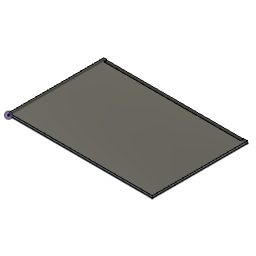
Clear Nomad 3 - Top Panel (Autodesk Fusion 360 design; units mm, degrees)
Autodesk Fusion 360 part; units mm, degrees
note: some values were not read from the file. Set by a fixed rule: which sketch regions a step uses.
sketch "Sketch1" plane through (0, 0, 0) normal (0, 0, 1) x (1, 0, 0)
  line L0 (0, 0) -> (417, 0)
  line L1 (417, 0) -> (417, 276)
  line L2 (0, 276) -> (0, 0)
  line L3 (0, 276) -> (417, 276)
  dimension "d1" = 417
  dimension "d2" = 276
  constraint horizontal L0
  constraint vertical L1
  constraint vertical L2
  constraint coincident L0.start L2.end
  constraint horizontal L3
  measures "d1" distance of L0.start L0.end
  measures "d2" distance of L0.start L2.start
extrude "Extrude1" add sketch "Sketch1" along normal blind 6
sketch "Sketch2" plane through (0, 0, 6) normal (0, 0, 1) x (-1, 0, 0)
  line L0 (0, 0) -> (-417, 0)
  line L1 (-417, 0) -> (-417, -276)
  line L2 (-417, -276) -> (0, -276)
  line L3 (0, -276) -> (0, 0)
  line L4 (-11, -276) -> (-406, -276)
  line L5 (-406, -276) -> (-406, -267)
  line L6 (-406, -267) -> (-11, -267)
  line L7 (-11, -267) -> (-11, -276)
  line L8 (-417, 0) -> (-417, -276)
  dimension "d8" = 9
  dimension "d9" = 395
  dimension "d12" = 11
  dimension "d13" = 11
  constraint horizontal L4
  constraint vertical L5
  constraint horizontal L6
  constraint vertical L7
  measures "d8" distance of L4.start L6.end
  measures "d9" distance of L4.start L4.end
  measures "d12" distance of L5 L8
  measures "d13" distance of L3 L7
extrude "Extrude3" cut sketch "Sketch2" against normal blind 1.2 contours L2 L4 L5 L6 L7
